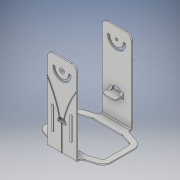
# Autodesk Inventor part: Drone_holder
Saved by Autodesk Inventor 2019 (Build 230136000, 136)
## iProperties
Created: 2020-01-23
Part Number: Drone_holder
Material: Generic
Document SubType Name: Modeling
Designer: Next
Density: 1 g/cm^3
Appearance: Default
Author: Next
## iProperties of the stored document Drone_holder_3DPrint.ipt
Created: 2020-01-25
Part Number: Drone_holder_3DPrint
Material: Generic
Document SubType Name: Modeling
Designer: Next
Density: 1 g/cm^3
Appearance: Default
Author: Next
Autodesk Inventor part; units mm, degrees
ref_plane "YZ Plane" through (0, 0, 0) normal (1, 0, 0) x (0, 1, 0)
ref_plane "XZ Plane" through (0, 0, 0) normal (0, 1, 0) x (-1, 0, 0)
ref_plane "XY Plane" through (0, 0, 0) normal (0, 0, 1) x (1, 0, 0)
sketch "Sketch1" plane through (0, 0, 0) normal (0, 1, 0) x (-1, 0, 0)
  line L0 (0, 0) -> (-140, 0) construction
  line L1 (-140, 0) -> (-140, -100) construction
  line L2 (-140, -100) -> (0, -100) construction
  line L3 (0, -100) -> (0, 0) construction
  line L4 (0, -50) -> (-140, -50) construction
  line L5 (-70, -100) -> (-70, 0) construction
  line L6 (-96.6886, -17.5) -> (-43.3114, -17.5) construction
  line L7 (-120, -71.3962) -> (-120, -28.6038) construction
  line L8 (-20, -28.6038) -> (-20, -71.3962) construction
  line L9 (-98.2698, -82.2434) -> (-116.5811, -76.1396)
  line L10 (-116.5811, -23.8604) -> (-98.2698, -17.7566)
  line L11 (-41.7302, -17.7566) -> (-23.4189, -23.8604)
  line L12 (-23.4189, -76.1396) -> (-41.7302, -82.2434)
  line L13 (-43.3114, -82.5) -> (-96.6886, -82.5)
  arc A0 (-23.4189, -76.1396) -> (-20, -71.3962) centre (-25, -71.3962) ccw
  arc A1 (-43.3114, -82.5) -> (-41.7302, -82.2434) centre (-43.3114, -77.5) ccw
  arc A2 (-98.2698, -82.2434) -> (-96.6886, -82.5) centre (-96.6886, -77.5) ccw
  arc A3 (-120, -71.3962) -> (-116.5811, -76.1396) centre (-115, -71.3962) ccw
  arc A4 (-116.5811, -23.8604) -> (-120, -28.6038) centre (-115, -28.6038) ccw
  arc A5 (-96.6886, -17.5) -> (-98.2698, -17.7566) centre (-96.6886, -22.5) ccw
  arc A6 (-41.7302, -17.7566) -> (-43.3114, -17.5) centre (-43.3114, -22.5) ccw
  arc A7 (-20, -28.6038) -> (-23.4189, -23.8604) centre (-25, -28.6038) ccw
  line L14 (-120, -71.3962) -> (-120, -28.6038)
  line L15 (-20, -28.6038) -> (-20, -71.3962)
  arc A8 (-101.432, -91.7302) -> (-100.4386, -92.0237) centre (-96.6886, -77.5) ccw
  line L16 (-101.432, -91.7302) -> (-119.7434, -85.6265)
  arc A9 (-130, -71.3962) -> (-119.7434, -85.6265) centre (-115, -71.3962) ccw
  line L17 (-130, -71.3962) -> (-130, -28.6038)
  arc A10 (-119.7434, -14.3735) -> (-130, -28.6038) centre (-115, -28.6038) ccw
  line L18 (-119.7434, -14.3735) -> (-101.432, -8.2698)
  arc A11 (-100.4386, -7.9763) -> (-101.432, -8.2698) centre (-96.6886, -22.5) ccw
  arc A12 (-38.568, -8.2698) -> (-39.5614, -7.9763) centre (-43.3114, -22.5) ccw
  line L19 (-38.568, -8.2698) -> (-20.2566, -14.3735)
  arc A13 (-10, -28.6038) -> (-20.2566, -14.3735) centre (-25, -28.6038) ccw
  line L20 (-10, -28.6038) -> (-10, -71.3962)
  arc A14 (-20.2566, -85.6265) -> (-10, -71.3962) centre (-25, -71.3962) ccw
  line L21 (-20.2566, -85.6265) -> (-38.568, -91.7302)
  arc A15 (-39.5614, -92.0237) -> (-38.568, -91.7302) centre (-43.3114, -77.5) ccw
  line L22 (-96.6886, -17.5) -> (-43.3114, -17.5)
  line L23 (-96.6886, -3.1351) -> (-96.6886, 1.5)
  line L24 (-96.6886, 1.5) -> (-43.3114, 1.5)
  line L25 (-43.3114, 1.5) -> (-43.3114, -3.1351)
  line L26 (-96.6886, -96.8649) -> (-96.6886, -101.5)
  line L27 (-96.6886, -101.5) -> (-43.3114, -101.5)
  line L28 (-43.3114, -101.5) -> (-43.3114, -96.8649)
  arc A16 (-96.6886, -96.8649) -> (-100.4386, -92.0237) centre (-101.6886, -96.8649) ccw
  arc A17 (-39.5614, -92.0237) -> (-43.3114, -96.8649) centre (-38.3114, -96.8649) ccw
  arc A18 (-43.3114, -3.1351) -> (-39.5614, -7.9763) centre (-38.3114, -3.1351) ccw
  arc A19 (-100.4386, -7.9763) -> (-96.6886, -3.1351) centre (-101.6886, -3.1351) ccw
  point P0 (-70, -50)
  dimension "d0" = 140
  dimension "d1" = 100
  dimension "d6" = 5
  dimension "d10" = 5
  constraints: 58 end point, 40 point on circle, 23 tangent, 20 centre point, 10 equal radius, 10 parallel, 5 midpoint, 3 horizontal, 2 perpendicular, 12 other
  measures "d0" distance of L2.end L1.end
  measures "d1" distance of L1.end L0.end
  measures "d6" radius of A0
  measures "d10" radius of A16
extrude "Extrusion1" add sketch "Sketch1" along normal blind 2
sketch "Sketch2" plane through (0, 2, 0) normal (0, 1, 0) x (1, 0, 0)
  line L0 (43.3114, 1) -> (96.6886, 1) construction
  line L1 (43.3114, 99) -> (96.6886, 99) construction
  line L2 (96.6886, 101.5) -> (43.3114, 101.5) construction
  line L3 (43.3114, -1.5) -> (96.6886, -1.5) construction
  line L4 (43.3114, -1.5) -> (96.6886, -1.5) projected
  line L5 (43.3114, 1) -> (96.6886, 1)
  line L6 (96.6886, 1) -> (96.6886, -1.5)
  line L7 (96.6886, -1.5) -> (43.3114, -1.5)
  line L8 (43.3114, -1.5) -> (43.3114, 1)
  line L9 (43.3114, 101.5) -> (96.6886, 101.5)
  line L10 (96.6886, 101.5) -> (96.6886, 99)
  line L11 (96.6886, 99) -> (43.3114, 99)
  line L12 (43.3114, 99) -> (43.3114, 101.5)
  point P0 (0, 0)
  dimension "d13" = 2.5
  dimension "d14" = 2.5
  constraints: 20 end point, 4 horizontal, 4 parallel, 2 perpendicular
  measures "d13" distance between parallel lines of L1 L2
  measures "d14" distance between parallel lines of L3 L0
extrude "Extrusion2" add sketch "Sketch2" along normal blind 150
fillet "Fillet1" radius 2 4 edges at (70, 2, -1) (70, 2, -99) (70, 0, 1.5) (70, 0, -101.5)
sketch "Sketch3" plane through (96.6886, 0, -101.5) normal (0, 0, -1) x (-1, 0, 0)
  line L0 (0, 2) -> (0, 152) construction
  line L1 (0, 132) -> (24.3997, 132) construction
  line L2 (0, 152) -> (53.3772, 152) construction
  circle A0 centre (26.6497, 132) radius 2.25
  line L3 (28.8997, 132) -> (53.2994, 132) construction
  line L4 (24.3997, 132) -> (28.8997, 132) construction
  circle A1 centre (41.0995, 132) radius 2.25
  circle A2 centre (12.1998, 132) radius 2.25
  arc A3 (9.9498, 132) -> (43.3495, 132) centre (26.6497, 132) ccw
  arc A4 (14.4498, 132) -> (38.8495, 132) centre (26.6497, 132) ccw
  arc A5 (14.4498, 132) -> (9.9498, 132) centre (12.1998, 132) ccw
  arc A6 (43.3495, 132) -> (38.8495, 132) centre (41.0995, 132) ccw
  point P0 (96.6886, 0)
  point P1 (0, 0)
  dimension "d19" = 4.5
  dimension "d20" = 4.5
  dimension "d21" = 4.5
  dimension "d42" = 4.5
  constraints: 10 point on circle, 7 centre point, 6 end point, 4 tangent, 3 horizontal, 2 midpoint, 1 point on line
  measures "d19" diameter of A0
  measures "d20" diameter of A1
  measures "d21" diameter of A2
  measures "d42" diameter of A6
extrude "Extrusion3" cut sketch "Sketch3" against normal blind 110
fillet "Fillet2" radius 10 4 edges at (43.3114, 152, -100.25) (96.6886, 152, -100.25) (43.3114, 152, 0.25) (96.6886, 152, 0.25)
sketch "Sketch4" plane through (96.6886, 0, -101.5) normal (0, 0, -1) x (-1, 0, 0)
  line L0 (0, 2) -> (53.3772, 2) construction
  line L1 (34.1886, 49) -> (19.1886, 49)
  line L2 (19.1886, 49) -> (19.1886, 57)
  line L3 (19.1886, 57) -> (34.1886, 57)
  line L4 (34.1886, 57) -> (34.1886, 49)
  point P0 (96.6886, 0)
  dimension "d26" = 15
  dimension "d27" = 8
  dimension "d28" = 47
  constraints: 8 end point, 2 parallel, 1 horizontal, 1 perpendicular
  measures "d26" distance of L2.end L3.end
  measures "d27" distance of L1.end L2.end
  measures "d28" distance between parallel lines of L1 L0
extrude "Extrusion4" cut sketch "Sketch4" against normal blind 110
fillet "Fillet3" radius 5 4 edges at (62.5, 57, -100.25) (77.5, 57, -100.25) (62.5, 57, 0.25) (77.5, 57, 0.25)
sketch "Sketch5" plane through (96.6886, 4, -1) normal (0, 0, -1) x (-1, 0, 0)
  line L0 (39.1886, 45) -> (14.1886, 45)
  line L1 (14.1886, 45) -> (14.1886, 43)
  line L2 (14.1886, 43) -> (39.1886, 43)
  line L3 (39.1886, 43) -> (39.1886, 45)
  line L4 (34.1886, 45) -> (19.1886, 45) projected
  point P0 (96.6886, -4)
  point P1 (26.6886, 44)
  dimension "d32" = 25
  dimension "d33" = 2
  constraints: 8 end point, 2 parallel, 1 horizontal, 1 perpendicular, 1 other
  measures "d32" distance of L2.end L1.end
  measures "d33" distance of L1.end L0.end
extrude "Extrusion5" add sketch "Sketch5" along normal blind 98
sketch "Sketch6" plane through (62.5, 49, -101.5) normal (0, 1, 0) x (1, 0, 0)
  line L0 (-5, -17.5) -> (20, -17.5)
  line L1 (20, -17.5) -> (20, -85.5)
  line L2 (20, -85.5) -> (-5, -85.5)
  line L3 (-5, -85.5) -> (-5, -17.5)
  line L4 (20, -100.5) -> (15, -100.5) construction
  line L5 (0, -100.5) -> (-5, -100.5) construction
  line L6 (20, -100.5) -> (-5, -100.5) construction
  line L7 (15, -2.5) -> (20, -2.5) construction
  line L8 (-5, -2.5) -> (0, -2.5) construction
  line L9 (20, -2.5) -> (-5, -2.5) construction
  point P0 (-62.5, -101.5)
  dimension "d37" = 15
  dimension "d38" = 15
  constraints: 12 end point, 2 horizontal, 2 parallel, 1 collinear, 1 perpendicular
  measures "d37" distance between parallel lines of L2 L6
  measures "d38" distance between parallel lines of L9 L0
extrude "Extrusion6" cut sketch "Sketch6" against normal blind 3
fillet "Fillet4" radius 5 10 edges at (70, 47, -1) (70, 47, -99) (80, 49, -99) (60, 49, -99) (80, 49, -1) (60, 49, -1) (82.5, 48, -16) (57.5, 48, -16) (82.5, 48, -84) (57.5, 48, -84)
sketch "Sketch8" plane through (96.6886, 2, -101.5) normal (0, 0, -1) x (-1, 0, 0)
  line L0 (53.3772, 2) -> (53.3772, 140) construction
  line L1 (53.3772, 110) -> (0, 110) construction
  line L2 (0, 2) -> (0, 140) construction
  line L3 (10, 150) -> (43.3772, 150) construction
  line L4 (53.3772, 0) -> (0, 0) construction
  line L5 (34.1886, 47) -> (19.1886, 47) construction
  line L6 (24.1886, 55) -> (29.1886, 55) construction
  arc A0 (24.1886, 55) -> (19.1886, 50) centre (24.1886, 50) ccw construction
  arc A1 (34.1886, 50) -> (29.1055, 55) centre (29.1876, 49.9996) ccw construction
  arc A2 (53.3772, 110) -> (30.6062, 54.7948) centre (206.0864, 14.7115) ccw construction
  arc A3 (52.953, 110.2647) -> (30.1201, 54.9125) centre (206.0864, 14.7115) ccw
  arc A4 (22.7711, 54.7948) -> (0, 110) centre (-152.7092, 14.7115) ccw construction
  arc A5 (22.2836, 54.6835) -> (0, 109.0521) centre (-152.7092, 14.7115) ccw
  arc A6 (22.2836, 54.6835) -> (22.2993, 54.6293) centre (22.7711, 54.7948) ccw
  arc A7 (0.4242, 110.2647) -> (0, 110.5) centre (0, 110) ccw
  line L7 (26.1886, 47) -> (26.1886, 0)
  line L8 (27.1886, 0) -> (27.1886, 47)
  line L9 (27.1886, 47) -> (26.1886, 47)
  line L10 (27.1886, 0) -> (26.1886, 0)
  arc A8 (31.0779, 54.6293) -> (31.0936, 54.6835) centre (30.6062, 54.7948) ccw
  arc A9 (31.0779, 54.6293) -> (30.1201, 54.9125) centre (29.1886, 50) ccw
  line L11 (53.3772, 109.0521) -> (53.3772, 110.5)
  arc A10 (53.3772, 109.0521) -> (31.0936, 54.6835) centre (206.0864, 14.7115) ccw
  arc A11 (53.3772, 110.5) -> (52.953, 110.2647) centre (53.3772, 110) ccw
  arc A12 (24.1886, 55) -> (19.1886, 50) centre (24.1886, 50) ccw projected
  arc A13 (23.2571, 54.9125) -> (22.2993, 54.6293) centre (24.1886, 50) ccw
  arc A14 (23.2571, 54.9125) -> (0.4242, 110.2647) centre (-152.7092, 14.7115) ccw
  line L12 (0, 109.0521) -> (0, 110.5)
  point P0 (96.6886, -2)
  point P1 (26.6886, 23.5)
  dimension "d43" = 40
  constraints: 33 point on circle, 16 end point, 14 centre point, 4 point on line, 2 collinear, 2 tangent, 1 horizontal, 1 parallel
  measures "d43" distance between parallel lines of L3 L1
extrude "Extrusion9" add sketch "Sketch8" along normal blind 1
sketch "Sketch9" plane through (43.3114, 2, 1.5) normal (0, 0, 1) x (1, 0, 0)
  line L0 (0, 0) -> (53.3772, 0) construction
  line L1 (34.1886, 47) -> (19.1886, 47) construction
  line L2 (27.1886, 0) -> (27.1886, 47)
  line L3 (26.1886, 47) -> (26.1886, 0)
  line L4 (27.1886, 0) -> (26.1886, 0)
  line L5 (53.3772, 2) -> (53.3772, 140) construction
  line L6 (53.3772, 110) -> (0, 110) construction
  line L7 (10, 150) -> (43.3772, 150) construction
  arc A0 (52.953, 110.2647) -> (30.1201, 54.9125) centre (206.0864, 14.7115) ccw
  arc A1 (22.2836, 54.6835) -> (0, 109.0521) centre (-152.7092, 14.7115) ccw
  arc A2 (22.2836, 54.6835) -> (22.2993, 54.6293) centre (22.7711, 54.7948) ccw
  arc A3 (0.4242, 110.2647) -> (0, 110.5) centre (0, 110) ccw
  arc A4 (53.3772, 109.0521) -> (31.0936, 54.6835) centre (206.0864, 14.7115) ccw
  arc A5 (53.3772, 110.5) -> (52.953, 110.2647) centre (53.3772, 110) ccw
  line L8 (0, 2) -> (0, 140) projected
  line L9 (0, 109.0521) -> (0, 110.5)
  arc A6 (24.1886, 55) -> (19.1886, 50) centre (24.1886, 50) ccw projected
  arc A7 (23.2571, 54.9125) -> (22.2993, 54.6293) centre (24.1886, 50) ccw
  arc A8 (34.1886, 50) -> (29.1886, 55) centre (29.1886, 50) ccw projected
  arc A9 (31.0779, 54.6293) -> (30.1201, 54.9125) centre (29.1886, 50) ccw
  arc A10 (31.0779, 54.6293) -> (31.0936, 54.6835) centre (30.6062, 54.7948) ccw
  arc A11 (23.2571, 54.9125) -> (0.4242, 110.2647) centre (-152.7092, 14.7115) ccw
  line L10 (53.3772, 109.0521) -> (53.3772, 110.5)
  line L11 (27.1886, 47) -> (26.1886, 47)
  line L12 (19.1886, 47) -> (34.1886, 47) projected
  point P0 (-43.3114, -2)
  point P1 (26.6886, 23.5)
  dimension "d50" = 40
  constraints: 26 point on circle, 14 end point, 10 centre point, 5 point on line, 2 collinear, 2 tangent, 1 horizontal, 1 parallel, 1 perpendicular
  measures "d50" distance between parallel lines of L7 L6
extrude "Extrusion10" add sketch "Sketch9" along normal blind 1
sketch "Sketch10" plane through (77.5, 49, -101.5) normal (0, 0, -1) x (-1, 0, 0)
  line L0 (-5, 0) -> (0, 0) construction
  line L1 (0, 0) -> (-19.1886, 0) construction
  line L2 (-19.1886, -47) -> (-19.1886, 62.0521) construction
  line L3 (15, 0) -> (34.1886, 0) construction
  line L4 (34.1886, -47) -> (34.1886, 62.0521) construction
  line L5 (-9.5943, 20) -> (-9.5943, -20) construction
  line L6 (-11.5943, 20) -> (-11.5943, -20)
  line L7 (-7.5943, -20) -> (-7.5943, 20)
  arc A0 (-7.5943, 20) -> (-11.5943, 20) centre (-9.5943, 20) ccw
  arc A1 (-11.5943, -20) -> (-7.5943, -20) centre (-9.5943, -20) ccw
  line L8 (-9.5943, 0) -> (30.4057, 0) construction
  line L9 (24.5943, 20) -> (24.5943, -20) construction
  line L10 (22.5943, 20) -> (22.5943, -20)
  line L11 (26.5943, -20) -> (26.5943, 20)
  arc A2 (26.5943, 20) -> (22.5943, 20) centre (24.5943, 20) ccw
  arc A3 (22.5943, -20) -> (26.5943, -20) centre (24.5943, -20) ccw
  point P0 (77.5, -49)
  point P1 (24.5943, 0)
  dimension "d63" = 20
  dimension "d64" = 90
  dimension "d65" = 4
  dimension "d66" = 20
  dimension "d67" = 4
  constraints: 22 end point, 8 point on circle, 8 tangent, 4 centre point, 4 midpoint, 3 perpendicular, 3 point on line, 2 horizontal, 2 parallel
  measures "d63" distance of L8.start L5.end
  measures "d64" angle of L5 L8
  measures "d65" diameter of A1
  measures "d66" distance of point (24.594, 0) L9.end
  measures "d67" diameter of A3
extrude "Extrusion11" add sketch "Sketch10" along normal blind 1
sketch "Sketch11" plane through (62.5, 49, 1.5) normal (0, 0, 1) x (1, 0, 0)
  line L0 (0, 0) -> (-5, 0) construction
  line L1 (0, 0) -> (-19.1886, 0) construction
  line L2 (-19.1886, -47) -> (-19.1886, 62.0521) construction
  line L3 (8, 0) -> (15, 0) construction
  line L4 (15, 0) -> (34.1886, 0) construction
  line L5 (34.1886, -47) -> (34.1886, 62.0521) construction
  line L6 (-9.5943, 20) -> (-9.5943, -20) construction
  line L7 (-11.5943, 20) -> (-11.5943, -20)
  line L8 (-7.5943, -20) -> (-7.5943, 20)
  arc A0 (-7.5943, 20) -> (-11.5943, 20) centre (-9.5943, 20) ccw
  arc A1 (-11.5943, -20) -> (-7.5943, -20) centre (-9.5943, -20) ccw
  line L9 (-9.5943, 0) -> (30.4057, 0) construction
  line L10 (24.5943, -20) -> (24.5943, 20) construction
  line L11 (26.5943, -20) -> (26.5943, 20)
  line L12 (22.5943, 20) -> (22.5943, -20)
  arc A2 (22.5943, -20) -> (26.5943, -20) centre (24.5943, -20) ccw
  arc A3 (26.5943, 20) -> (22.5943, 20) centre (24.5943, 20) ccw
  line L13 (24.5943, 0) -> (64.5943, 0) construction
  point P0 (-62.5, -49)
  dimension "d70" = 20
  dimension "d71" = 90
  dimension "d72" = 4
  dimension "d73" = 20
  dimension "d74" = 90
  dimension "d75" = 4
  constraints: 24 end point, 8 point on circle, 8 tangent, 4 centre point, 4 midpoint, 4 perpendicular, 3 horizontal, 3 point on line, 2 parallel
  measures "d70" distance of L9.start L6.end
  measures "d71" angle of L6 L9
  measures "d72" diameter of A1
  measures "d73" distance of L13.start L10.end
  measures "d74" angle of L13 L10
  measures "d75" diameter of A3
extrude "Extrusion12" add sketch "Sketch11" along normal blind 1
sketch "Sketch12" plane through (53.3114, 152, 1.5) normal (0, 0, 1) x (1, 0, 0)
  circle A0 centre (16.7291, -20.0013) radius 4.6
  point P0 (-53.3114, -152)
  dimension "d78" = 9.2
  constraints: 1 centre point
  measures "d78" diameter of A0
extrude "Extrusion13" cut sketch "Sketch12" against normal blind 0.1
sketch "Sketch13" plane through (86.6886, 152, -101.5) normal (0, 0, -1) x (-1, 0, 0)
  circle A0 centre (16.6589, -19.9967) radius 4.6
  point P0 (86.6886, -152)
  dimension "d81" = 9.2
  constraints: 1 centre point
  measures "d81" diameter of A0
extrude "Extrusion14" cut sketch "Sketch13" against normal blind 0.1
sketch "Sketch7" plane through (43.3114, 2, 1.5) normal (0, 0, 1) x (1, 0, 0)
  circle A0 centre (26.7275, 130) radius 2.25 projected
  arc A1 (43.4274, 130) -> (38.9274, 130) centre (41.1774, 130) ccw projected
  arc A2 (14.5277, 130) -> (10.0277, 130) centre (12.2777, 130) ccw projected
  arc A3 (12.2777, 130) -> (41.1774, 130) centre (26.7275, 130) ccw construction
  arc A4 (10.0277, 130) -> (43.4274, 130) centre (26.7275, 130) ccw
  arc A5 (14.5277, 130) -> (38.9274, 130) centre (26.7275, 130) ccw
  arc A6 (14.5277, 130) -> (10.0277, 130) centre (12.2777, 130) ccw
  arc A7 (43.4274, 130) -> (38.9274, 130) centre (41.1774, 130) ccw
  point P0 (-43.3114, -2)
  constraints: 10 point on circle, 5 centre point, 4 tangent, 3 coincident, 1 concentric
body "Solid1"
